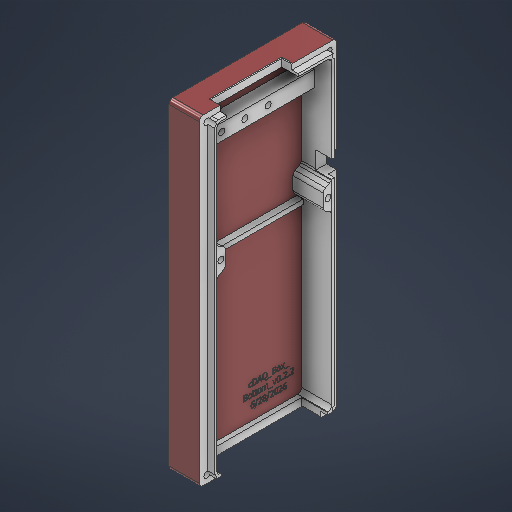
# Autodesk Inventor part: cDAQ_Box_Bottom_v0.2.3
Saved by Autodesk Inventor 2027 (Build 310192000, 192)
## iProperties
Created: 2026-05-08
Part Number: cDAQ_Box_Bottom_v0.2.3
Material: Generic
Document SubType Name: Modeling
Designer: giese
Density: 1 g/cm^3
Appearance: Default
Author: giese
Autodesk Inventor part; units mm, degrees
(part 1 of 2)
ref_plane "YZ Plane" through (0, 0, 0) normal (1, 0, 0) x (0, 1, 0)
ref_plane "XZ Plane" through (0, 0, 0) normal (0, 1, 0) x (-1, 0, 0)
ref_plane "XY Plane" through (0, 0, 0) normal (0, 0, 1) x (1, 0, 0)
sketch "Sketch1" plane through (0, 0, 0) normal (1, 0, 0) x (0, 1, 0)
  line L0 (37.5698, 60.7867) -> (-217.4462, 60.7867)
  line L1 (-217.4462, 60.7867) -> (-217.4462, -48.4333)
  line L2 (-217.4462, -48.4333) -> (37.5698, -48.4333)
  line L3 (37.5698, -48.4333) -> (37.5698, 60.7867)
  point P0 (0, 0)
  dimension "d0" = 109.22
  dimension "d1" = 255.016
  constraints: 8 end point, 2 parallel, 1 horizontal, 1 perpendicular
  measures "d0" distance of L2.end L0.start
  measures "d1" distance of L1.end L2.end
extrude "Extrusion1" add sketch "Sketch1" along normal blind 24.13
sketch "Sketch2" plane through (24.13, 0, 0) normal (1, 0, 0) x (0, 0, -1)
  line L0 (39.5433, 31.2198) -> (-51.8967, 31.2198)
  line L1 (-51.8967, 31.2198) -> (-51.8967, -211.0962)
  line L2 (-51.8967, -211.0962) -> (39.5433, -211.0962)
  line L3 (39.5433, -211.0962) -> (39.5433, 31.2198)
  line L4 (48.4333, 37.5698) -> (-60.7867, 37.5698) projected
  line L5 (-60.7867, 37.5698) -> (-60.7867, -217.4462) projected
  line L6 (-60.7867, -217.4462) -> (48.4333, -217.4462) projected
  line L7 (48.4333, -217.4462) -> (48.4333, 37.5698) projected
  point P0 (0, 0)
  dimension "d4" = 242.316
  dimension "d5" = 91.44
  dimension "d8" = 6.35
  dimension "d21" = 8.89
  dimension "d690" = 6.35
  dimension "d842" = 8.89
  constraints: 8 end point, 2 parallel, 1 horizontal, 1 perpendicular
  measures "d4" distance of L2.end L0.start
  measures "d5" distance of L0.start L0.end
  measures "d8" distance between parallel lines of L0 L4
  measures "d21" distance between parallel lines of L5 L1
  measures "d690" distance between parallel lines of L6 L2
  measures "d842" distance between parallel lines of L7 L3
extrude "Extrusion2" cut sketch "Sketch2" against normal blind 19.05 contours L3 L2 L1 L0
sketch "Sketch3" plane through (0, 0, 0) normal (-1, 0, 0) x (0, 0, 1)
  circle A0 centre (-2.8809, 9.6298) radius 2.4005
  circle A1 centre (15.6179, 9.6298) radius 2.4005
  circle A2 centre (34.1167, 9.6298) radius 2.4005
  line L0 (-48.4333, -217.4462) -> (-48.4333, 37.5698) projected
  line L1 (-48.4333, 37.5698) -> (60.7867, 37.5698) projected
  line L2 (60.7867, 37.5698) -> (60.7867, -217.4462) projected
  line L3 (51.8967, 31.2198) -> (-39.5433, 31.2198) projected
  point P0 (0, 0)
  point P1 (-0.896, -23.7433)
  point P2 (-45.1848, 27.0137)
  dimension "d9" = 18.4988
  dimension "d10" = 4.801
  dimension "d11" = 4.801
  dimension "d12" = 18.4988
  dimension "d13" = 36.9976
  dimension "d18" = 26.67
  dimension "d22" = 4.801
  dimension "d58" = 27.94
  constraints: 3 centre point
  measures "d9" distance of A0.centre A1.centre
  measures "d10" diameter of A1
  measures "d11" diameter of A2
  measures "d12" distance of A1.centre A2.centre
  measures "d13" distance of A0.centre A2.centre
  measures "d18" distance from line of L2 A2.centre
  measures "d22" diameter of A0
  measures "d58" distance from line of L1 A2.centre
extrude "Extrusion3" cut sketch "Sketch3" against normal blind 5.08
sketch "Sketch5" plane through (0, -217.4462, -48.4333) normal (0, 0, -1) x (-1, 0, 0)
  line L0 (-27.2034, 165.862) -> (-16.51, 165.862)
  line L1 (-16.51, 165.862) -> (-16.51, 178.562)
  line L2 (-16.51, 178.562) -> (-27.2034, 178.562)
  line L3 (-27.2034, 178.562) -> (-27.2034, 165.862)
  line L4 (0, 255.016) -> (-24.13, 255.016) projected
  line L5 (0, 0) -> (0, 255.016) projected
  line L6 (-24.13, 0) -> (-24.13, 255.016) projected
  line L7 (0, 0) -> (-24.13, 0) projected
  point P0 (0, 217.4462)
  point P1 (-21.8567, 178.562)
  point P2 (-21.8567, 165.862)
  dimension "d28" = 10.6934
  dimension "d30" = 12.7
  dimension "d31" = 16.51
  dimension "d215" = 3.0734
  dimension "d1133" = 165.862
  constraints: 8 end point, 2 midpoint, 2 parallel, 1 horizontal, 1 perpendicular
  measures "d28" distance between parallel lines of L1 L3
  measures "d30" distance of point (-21.857, 178.562) point (-21.857, 165.862)
  measures "d31" distance between parallel lines of L5 L1
  measures "d215" distance between parallel lines of L6 L3
  measures "d1133" distance between parallel lines of L7 L0
extrude "Extrusion4" cut sketch "Sketch5" against normal blind 24.13 contours L3 L2 L6 L0 | L6 L2 L1 L0
sketch "Sketch6" plane through (0, -217.4462, -48.4333) normal (0, -1, 0) x (1, 0, 0)
  line L0 (24.08, 55.136) -> (16.08, 55.136)
  line L1 (16.08, 45.136) -> (24.08, 45.136)
  line L2 (0, 109.22) -> (0, 0) projected
  line L3 (29.63, 53.1359) -> (29.63, 47.136)
  line L4 (24.08, 55.136) -> (29.63, 53.1359)
  line L5 (29.63, 47.136) -> (24.08, 45.136)
  line L6 (0, 0) -> (24.13, 0) projected
  line L7 (24.13, 100.33) -> (24.13, 8.89) projected
  line L8 (24.13, 41.9134) -> (24.13, 37.4697)
  line L9 (16.08, 55.136) -> (8.636, 55.136)
  line L10 (8.636, 55.136) -> (8.636, 45.136)
  line L11 (8.636, 45.136) -> (21.16, 45.136)
  point P0 (0, 48.4333)
  point P1 (20.08, 55.136)
  point P2 (20.08, 45.136)
  point P3 (16.08, 50.136)
  dimension "d39" = 6
  dimension "d48" = 55.136
  dimension "d221" = 0
  dimension "d223" = 2
  dimension "d224" = 2
  dimension "d225" = 5.5
  dimension "d227" = 5.55
  dimension "d672" = 8.636
  constraints: 18 end point, 2 horizontal, 2 midpoint, 2 parallel, 2 point on line, 1 perpendicular, 1 vertical
  measures "d39" distance of L3.start L3.end
  measures "d48" distance between parallel lines of L6 L0
  measures "d221" horizontal distance of L0.start L1.end
  measures "d223" vertical distance of L3.end L1.end
  measures "d224" vertical distance of L0.start L3.start
  measures "d225" distance between parallel lines of L3 L7
  measures "d227" distance from line of L1.end L3
  measures "d672" distance between parallel lines of L2 L10
extrude "Extrusion5" [suppressed]
sketch "Sketch7" plane through (0, 37.5698, 60.7867) normal (0, 1, 0) x (1, 0, 0)
  line L0 (31.0134, 73.66) -> (16.002, 73.66)
  line L1 (16.002, 73.66) -> (16.002, 16.51)
  line L2 (16.002, 16.51) -> (31.0134, 16.51)
  line L3 (31.0134, 16.51) -> (31.0134, 73.66)
  line L4 (0, 0) -> (24.13, 0) projected
  line L5 (0, 109.22) -> (0, 0) projected
  line L6 (24.13, 109.22) -> (24.13, 0) projected
  point P0 (0, 60.7867)
  point P1 (24.13, 73.66)
  point P2 (24.13, 16.51)
  dimension "d52" = 16.51
  dimension "d55" = 16.002
  dimension "d56" = 15.0114
  dimension "d57" = 6.8834
  dimension "d1702" = 57.15
  constraints: 8 end point, 2 parallel, 1 horizontal, 1 perpendicular
  measures "d52" distance between parallel lines of L4 L2
  measures "d55" distance between parallel lines of L5 L1
  measures "d56" distance between parallel lines of L3 L1
  measures "d57" distance between parallel lines of L6 L3
  measures "d1702" distance of L2.end L0.start
extrude "Extrusion6" cut sketch "Sketch7" against normal blind 7.62
fillet "Fillet1" radius 3.175 4 edges at (12.065, 37.5698, -48.4333) (12.065, 37.5698, 60.7867) (12.065, -217.4462, -48.4333) (12.065, -217.4462, 60.7867)
sketch "Sketch8" plane through (0, 0, 0) normal (-1, 0, 0) x (0, 0, 1)
  line L0 (13.7764, 5.9468) -> (17.4594, 5.9468)
  line L1 (13.7764, 13.3128) -> (17.4594, 13.3128)
  line L2 (13.7764, 5.9468) -> (11.65, 9.6298)
  line L3 (13.7764, 13.3128) -> (11.65, 9.6298)
  line L4 (17.4594, 5.9468) -> (19.5858, 9.6298)
  line L5 (17.4594, 13.3128) -> (19.5858, 9.6298)
  circle A0 centre (15.6179, 9.6298) radius 2.4005
  circle A1 centre (15.6179, 9.6298) radius 2.4005 projected
  line L6 (-1.0394, 13.3128) -> (1.0869, 9.6298)
  line L7 (-1.0394, 5.9468) -> (1.0869, 9.6298)
  line L8 (-4.7224, 13.3128) -> (-1.0394, 13.3128)
  line L9 (-4.7224, 5.9468) -> (-1.0394, 5.9468)
  circle A2 centre (-2.8809, 9.6298) radius 2.4005
  line L10 (-4.7224, 13.3128) -> (-6.8488, 9.6298)
  line L11 (-4.7224, 5.9468) -> (-6.8488, 9.6298)
  circle A3 centre (-2.8809, 9.6298) radius 2.4005
  circle A4 centre (-2.8809, 9.6298) radius 2.4005 projected
  line L12 (35.9582, 13.3128) -> (38.0846, 9.6298)
  line L13 (35.9582, 5.9468) -> (38.0846, 9.6298)
  line L14 (32.2752, 13.3128) -> (35.9582, 13.3128)
  line L15 (32.2752, 5.9468) -> (35.9582, 5.9468)
  circle A5 centre (34.1167, 9.6298) radius 2.4005
  line L16 (32.2752, 13.3128) -> (30.1488, 9.6298)
  line L17 (32.2752, 5.9468) -> (30.1488, 9.6298)
  circle A6 centre (34.1167, 9.6298) radius 2.4005
  circle A7 centre (34.1167, 9.6298) radius 2.4005 projected
  point P0 (15.6179, 5.9468)
  point P1 (-2.8809, 5.9468)
  point P2 (34.1167, 5.9468)
  point P3 (1.0869, 9.6298)
  dimension "d1514" = 120
  dimension "d1515" = 120
  dimension "d1516" = 120
  dimension "d1517" = 120
  dimension "d1518" = 3.683
  dimension "d1519" = 3.683
  dimension "d1520" = 3.683
  dimension "d1521" = 3.683
  dimension "d1522" = 0
  dimension "d1523" = 3.683
  dimension "d1524" = 0
  dimension "d1525" = 3.683
  dimension "d1526" = 1.8415
  dimension "d1527" = 7.366
  dimension "d1528" = 7.9358
  dimension "d1529" = 0
  dimension "d1530" = 0
  dimension "d1531" = 7.9358
  dimension "d1532" = 0
  dimension "d1710" = 120
  dimension "d1711" = 120
  dimension "d1712" = 120
  dimension "d1713" = 120
  dimension "d1714" = 3.683
  dimension "d1715" = 3.683
  dimension "d1716" = 3.683
  dimension "d1717" = 3.683
  dimension "d1718" = 0
  dimension "d1719" = 3.683
  dimension "d1720" = 0
  dimension "d1721" = 3.683
  dimension "d1722" = 1.8415
  dimension "d1723" = 7.366
  dimension "d1724" = 7.9358
  dimension "d1725" = 0
  dimension "d1726" = 0
  dimension "d1727" = 7.9358
  dimension "d1728" = 0
  dimension "d1729" = 0
  dimension "d1730" = 0
  dimension "d1731" = 120
  dimension "d1732" = 120
  dimension "d1733" = 120
  dimension "d1734" = 120
  dimension "d1735" = 3.683
  dimension "d1736" = 3.683
  dimension "d1737" = 3.683
  dimension "d1738" = 3.683
  dimension "d1739" = 0
  dimension "d1740" = 3.683
  dimension "d1741" = 0
  dimension "d1742" = 3.683
  dimension "d1743" = 1.8415
  dimension "d1744" = 7.366
  dimension "d1745" = 7.9358
  dimension "d1746" = 0
  dimension "d1747" = 0
  dimension "d1748" = 7.9358
  dimension "d1749" = 0
  dimension "d1750" = 0
  dimension "d1751" = 0
  constraints: 36 end point, 6 horizontal, 5 centre point, 3 midpoint
  measures "d1514" angle of L0 L2
  measures "d1515" angle of L1 L3
  measures "d1516" angle of L4 L0
  measures "d1517" angle of L5 L1
  measures "d1518" distance of L0.start L4.start
  measures "d1519" distance of L1.start L5.start
  measures "d1520" vertical distance of L4.start L4.end
  measures "d1521" vertical distance of L3.end L1.start
  measures "d1522" vertical distance of A0.centre L3.end
  measures "d1523" vertical distance of L2.end L0.start
  measures "d1524" vertical distance of A0.centre L2.end
  measures "d1525" vertical distance of L5.end L5.start
  measures "d1526" horizontal distance of A0.centre L5.start
  measures "d1527" distance of L4.start L5.start
  measures "d1528" distance of L3.end L5.end
  measures "d1529" distance of A1.centre A0.centre
  measures "d1530" distance of A1.centre A0.centre
  measures "d1531" distance of L4.end L2.end
  measures "d1532" distance of L3.end L2.end
  measures "d1710" angle of L9 L11
  measures "d1711" angle of L8 L10
  measures "d1712" angle of L7 L9
  measures "d1713" angle of L6 L8
  measures "d1714" distance of L9.start L9.end
  measures "d1715" distance of L10.start L6.start
  measures "d1716" vertical distance of L9.end L7.end
  measures "d1717" vertical distance of L10.end L10.start
  measures "d1718" vertical distance of A2.centre L10.end
  measures "d1719" vertical distance of L11.end L9.start
  measures "d1720" vertical distance of A2.centre L11.end
  measures "d1721" vertical distance of L6.end L6.start
  measures "d1722" horizontal distance of A2.centre L6.start
  measures "d1723" distance of L9.end L6.start
  measures "d1724" distance of L10.end L6.end
  measures "d1725" distance of A3.centre A2.centre
  measures "d1726" distance of A3.centre A2.centre
  measures "d1727" distance of L7.end L11.end
  measures "d1728" distance of L10.end L11.end
  measures "d1729" distance of A4.centre A2.centre
  measures "d1730" distance of A4.centre A3.centre
  measures "d1731" angle of L15 L17
  measures "d1732" angle of L14 L16
  measures "d1733" angle of L13 L15
  measures "d1734" angle of L12 L14
  measures "d1735" distance of L17.start L13.start
  measures "d1736" distance of L16.start L12.start
  measures "d1737" vertical distance of L13.start L13.end
  measures "d1738" vertical distance of L16.end L16.start
  measures "d1739" vertical distance of A5.centre L16.end
  measures "d1740" vertical distance of L17.end L17.start
  measures "d1741" vertical distance of A5.centre L17.end
  measures "d1742" vertical distance of L12.end L12.start
  measures "d1743" horizontal distance of A5.centre L12.start
  measures "d1744" distance of L13.start L12.start
  measures "d1745" distance of L16.end L12.end
  measures "d1746" distance of A6.centre A5.centre
  measures "d1747" distance of A6.centre A5.centre
  measures "d1748" distance of L13.end L17.end
  measures "d1749" distance of L16.end L17.end
  measures "d1750" distance of A7.centre A5.centre
  measures "d1751" distance of A7.centre A5.centre
extrude "Extrusion7" cut sketch "Sketch8" against normal blind 5
sketch "Sketch9" plane through (5.08, 0, 0) normal (1, 0, 0) x (0, 0, -1)
  arc A0 (22.2689, -180.8044) -> (16.8127, -180.8044) centre (19.5408, -178.3302) ccw
  line L0 (45.2583, 37.5698) -> (12.8733, 37.5698) projected
  line L1 (39.5433, 31.2198) -> (39.5433, -38.8842) projected
  arc A1 (17.6358, -185.9502) -> (21.4458, -185.9502) centre (19.5408, -185.9502) ccw
  line L2 (21.4458, -185.9502) -> (21.4458, -182.9374)
  line L3 (17.6358, -185.9502) -> (17.6358, -182.9374)
  arc A2 (22.2689, -180.8044) -> (21.4458, -182.9374) centre (24.6208, -182.9374) ccw
  arc A3 (17.6358, -182.9374) -> (16.8127, -180.8044) centre (14.4608, -182.9374) ccw
  arc A4 (-28.5311, -180.8044) -> (-33.9873, -180.8045) centre (-31.2592, -178.3302) ccw
  arc A5 (-33.1642, -185.9366) -> (-29.3542, -185.9502) centre (-31.2592, -185.9502) ccw
  line L4 (-29.3542, -185.9502) -> (-29.3542, -182.9374)
  line L5 (-33.1642, -185.9366) -> (-33.1642, -182.9374)
  arc A6 (-28.5311, -180.8044) -> (-29.3542, -182.9374) centre (-26.1792, -182.9374) ccw
  arc A7 (-33.1642, -182.9374) -> (-33.9873, -180.8045) centre (-36.3392, -182.9374) ccw
  line L6 (-44.2767, 37.5698) -> (-57.6117, 37.5698) projected
  line L7 (-51.8967, -211.0962) -> (-51.8967, 31.2198) projected
  point P0 (0, 0)
  point P1 (39.5433, -211.0962)
  point P2 (21.4458, -181.4823)
  point P3 (17.6358, -181.4823)
  point P4 (-29.3542, -181.4823)
  point P5 (-33.1642, -181.4823)
  point P6 (-51.8967, 31.2198)
  point P7 (-49.3567, -207.2862)
  dimension "d112" = 215.9
  dimension "d114" = 7.366
  dimension "d116" = 3.81
  dimension "d117" = 223.52
  dimension "d118" = 3.175
  dimension "d119" = 7.366
  dimension "d120" = 3.81
  dimension "d121" = 3.175
  dimension "d122" = 215.9
  dimension "d123" = 223.52
  dimension "d125" = 0
  dimension "d128" = 50.8
  dimension "d129" = 20.0025
  dimension "d130" = 0
  constraints: 20 point on circle, 8 centre point, 8 end point, 8 tangent, 4 point on line, 2 equal radius, 2 parallel, 2 vertical, 1 other
  measures "d112" distance from line of L0 A0.centre
  measures "d114" diameter of A0
  measures "d116" diameter of A1
  measures "d117" distance from line of L0 A1.centre
  measures "d118" radius of A2
  measures "d119" diameter of A4
  measures "d120" diameter of A5
  measures "d121" radius of A6
  measures "d122" distance from line of A4.centre L6
  measures "d123" distance from line of L6 A5.centre
  measures "d125" horizontal distance of A5.centre A4.centre
  measures "d128" distance of A5.centre A1.centre
  measures "d129" distance from line of L1 A0.centre
  measures "d130" horizontal distance of A0.centre A1.centre
extrude "Extrusion8" [suppressed]
sketch "Sketch10" plane through (24.13, 0, 0) normal (1, 0, 0) x (0, 0, -1)
  line L0 (-51.8967, 31.2198) -> (39.5433, 31.2198) projected
  line L1 (-51.8967, 31.2198) -> (39.5433, 31.2198)
  line L2 (42.0833, 33.2264) -> (-46.8167, 33.2264)
  line L3 (-46.8167, 33.2264) -> (-53.9033, 33.2264)
  line L4 (-53.9033, 33.2264) -> (-53.9033, -213.1028)
  line L5 (-53.9033, -213.1028) -> (41.5499, -213.1028)
  line L6 (41.5499, -213.1028) -> (41.5499, 33.2264)
  line L7 (41.5499, 33.2264) -> (41.9392, 33.2264)
  line L8 (39.5433, 31.2198) -> (39.5433, -38.8842) projected
  line L9 (-51.8967, -211.0962) -> (-51.8967, 31.2198) projected
  line L10 (39.5433, -211.0962) -> (-51.8967, -211.0962) projected
  line L11 (45.2583, 37.5698) -> (12.8733, 37.5698) projected
  line L12 (39.5433, 31.2198) -> (39.5433, -211.0962)
  line L13 (39.5433, -211.0962) -> (-51.8967, -211.0962)
  line L14 (-57.6117, -217.4462) -> (45.2583, -217.4462) projected
  line L15 (-51.8967, -211.0962) -> (-51.8967, 31.2198)
  line L16 (-51.8967, 31.2198) -> (39.5433, 31.2198)
  line L17 (-51.8967, 31.2198) -> (39.5433, 31.2198)
  line L18 (39.5433, 31.2198) -> (39.5433, -211.0962)
  line L19 (39.5433, -211.0962) -> (-51.8967, -211.0962)
  line L20 (-51.8967, -211.0962) -> (-51.8967, 31.2198)
  point P0 (41.5499, 33.2264)
  point P1 (-49.3567, -207.2862)
  point P2 (39.5433, -38.8842)
  dimension "d202" = 2.0066
  dimension "d203" = 2.0066
  dimension "d204" = 2.0066
  dimension "d205" = 2.0066
  dimension "d208" = 4.3434
  constraints: 30 end point, 6 perpendicular, 3 collinear, 3 point on line, 2 horizontal, 2 parallel, 2 other
  measures "d202" distance between parallel lines of L0 L2
  measures "d203" distance between parallel lines of L6 L8
  measures "d205" distance between parallel lines of L5 L10
  measures "d208" distance between parallel lines of L11 L2
extrude "Extrusion9" add sketch "Sketch10" along normal blind 5
fillet "Fillet2" radius 3.175 7 edges at (17.105, 31.2198, -39.5433) (17.105, 31.2198, 51.8967) (17.105, -211.0962, 51.8967) (17.105, -211.0962, -39.5433) (26.63, 33.2264, 53.9033) (26.63, -213.1028, -41.5499) (26.63, -213.1028, 53.9033)
sketch "Sketch13" plane through (29.13, 0, 0) normal (1, 0, 0) x (0, 0, -1)
  arc A0 (44.0833, 30.0448) -> (40.9083, 33.2198) centre (40.9083, 30.0448) ccw projected
  arc A1 (-45.6417, 33.2198) -> (-48.8167, 30.0448) centre (-45.6417, 30.0448) ccw projected
  arc A2 (40.9083, -212.0802) -> (44.0833, -208.9052) centre (40.9083, -208.9052) ccw projected
  arc A3 (-48.8167, -208.9052) -> (-45.6417, -212.0802) centre (-45.6417, -208.9052) ccw projected
  line L0 (-44.2767, 37.5698) -> (-57.6117, 37.5698) projected
  line L1 (-60.7867, 34.3948) -> (-60.7867, -214.2712) projected
  line L2 (-57.6117, -217.4462) -> (45.2583, -217.4462) projected
  arc A4 (-48.8167, -208.9052) -> (-45.6417, -212.0802) centre (-45.6417, -208.9052) ccw projected
  circle A5 centre (-54.6907, -211.3502) radius 2.4005
  circle A6 centre (42.3373, -211.3502) radius 2.4005
  line L3 (48.4333, -214.2712) -> (48.4333, 34.3948) projected
  circle A7 centre (42.3373, 31.4738) radius 2.4005
  line L4 (45.2583, 37.5698) -> (12.8733, 37.5698) projected
  circle A8 centre (-54.6907, 31.4738) radius 2.4005
  arc A9 (41.4904, -28.6131) -> (38.3154, -25.4381) centre (38.3154, -28.6131) ccw
  circle A10 centre (36.3683, -64.0302) radius 2.4005
  circle A11 centre (-48.7217, -64.0302) radius 2.4005
  point P0 (0, 0)
  point P1 (-47.8868, 32.2898)
  point P2 (-47.8868, -211.1503)
  point P3 (-47.8868, -211.1503)
  point P4 (45.8404, -24.2631)
  point P5 (42.6654, -21.0881)
  dimension "d178" = 6.096
  dimension "d179" = 6.096
  dimension "d180" = 4.801
  dimension "d181" = 6.096
  dimension "d182" = 6.096
  dimension "d183" = 4.801
  dimension "d184" = 4.801
  dimension "d185" = 6.096
  dimension "d186" = 6.096
  dimension "d187" = 4.801
  dimension "d188" = 6.096
  dimension "d189" = 6.096
  dimension "d326" = 4.801
  dimension "d327" = 12.065
  dimension "d328" = 101.6
  dimension "d329" = 4.801
  dimension "d330" = 12.065
  dimension "d331" = 101.6
  constraints: 7 centre point, 5 point on circle
  measures "d178" distance from line of L1 A5.centre
  measures "d179" distance from line of L2 A5.centre
  measures "d180" diameter of A5
  measures "d181" distance from line of L2 A6.centre
  measures "d182" distance from line of L3 A6.centre
  measures "d183" diameter of A6
  measures "d184" diameter of A7
  measures "d185" distance from line of L3 A7.centre
  measures "d186" distance from line of L4 A7.centre
  measures "d187" diameter of A8
  measures "d188" distance from line of L0 A8.centre
  measures "d189" distance from line of L1 A8.centre
  measures "d326" diameter of A10
  measures "d327" distance from line of L3 A10.centre
  measures "d328" distance from line of A10.centre L4
  measures "d329" diameter of A11
  measures "d330" distance from line of L1 A11.centre
  measures "d331" distance from line of L0 A11.centre
extrude "Extrusion11" cut sketch "Sketch13" against normal blind 25.4
sketch "Sketch14" plane through (5.08, 0, 0) normal (1, 0, 0) x (0, 0, -1)
  line L0 (3.8756, -183.0595) -> (23.0923, -183.0595) construction
  line L1 (23.0923, -183.0595) -> (23.0923, -181.11) construction
  line L2 (23.0923, -181.11) -> (3.8756, -181.11) construction
  line L3 (3.8756, -181.11) -> (3.8756, -183.0595) construction
  spline S0 degree 2 poles (-1.0212, -187.8056) (-1.3769, -187.8056) (-1.966, -187.587) (-2.1772, -187.3647) knots 0 0 0 1 2 2 2
  spline S1 degree 2 poles (-2.1772, -187.3647) (-2.3884, -187.1461) (-2.6218, -186.4718) (-2.6218, -186.0198) knots 0 0 0 1 2 2 2
  spline S2 degree 2 poles (-2.6218, -186.0198) (-2.6218, -185.5678) (-2.381, -184.9083) (-2.1772, -184.686) knots 0 0 0 1 2 2 2
  spline S3 degree 2 poles (-2.1772, -184.686) (-1.9734, -184.46) (-1.3695, -184.2192) (-1.0212, -184.2192) knots 0 0 0 1 2 2 2
  spline S4 degree 2 poles (-1.0212, -184.2192) (-0.7396, -184.2192) (-0.2135, -184.3785) (-0.0097, -184.4822) knots 0 0 0 1 2 2 2
  line L4 (-0.0097, -184.4822) -> (-0.0097, -185.1306)
  line L5 (-0.0097, -185.1306) -> (-0.0431, -185.1306)
  spline S5 degree 2 poles (-0.0431, -185.1306) (-0.1061, -185.0787) (-0.2987, -184.9453) (-0.4358, -184.875) knots 0 0 0 1 2 2 2
  spline S6 degree 2 poles (-0.4358, -184.875) (-0.5581, -184.8157) (-0.8841, -184.723) (-1.0323, -184.723) knots 0 0 0 1 2 2 2
  spline S7 degree 2 poles (-1.0323, -184.723) (-1.4806, -184.723) (-2.0253, -185.4011) (-2.0253, -186.0198) knots 0 0 0 1 2 2 2
  spline S8 degree 2 poles (-2.0253, -186.0198) (-2.0253, -186.6237) (-1.4992, -187.3017) (-1.0323, -187.3017) knots 0 0 0 1 2 2 2
  spline S9 degree 2 poles (-1.0323, -187.3017) (-0.7507, -187.3017) (-0.2395, -187.0683) (-0.0431, -186.8868) knots 0 0 0 1 2 2 2
  line L6 (-0.0431, -186.8868) -> (-0.0097, -186.8868)
  line L7 (-0.0097, -186.8868) -> (-0.0097, -187.5352)
  spline S10 degree 2 poles (-0.0097, -187.5352) (-0.095, -187.5759) (-0.3543, -187.6908) (-0.4581, -187.7167) knots 0 0 0 1 2 2 2
  spline S11 degree 2 poles (-0.4581, -187.7167) (-0.6063, -187.7612) (-0.8397, -187.8056) (-1.0212, -187.8056) knots 0 0 0 1 2 2 2
  spline S12 degree 2 poles (4.1658, -185.4455) (4.1658, -186.0717) (3.6582, -187.0794) (3.2322, -187.361) knots 0 0 0 1 2 2 2
  spline S13 degree 2 poles (3.2322, -187.361) (2.8839, -187.5796) (2.1688, -187.7278) (1.6131, -187.7278) knots 0 0 0 1 2 2 2
  line L8 (1.6131, -187.7278) -> (0.5608, -187.7278)
  line L9 (0.5608, -187.7278) -> (0.5608, -183.1558)
  line L10 (0.5608, -183.1558) -> (1.6019, -183.1558)
  spline S14 degree 2 poles (1.6019, -183.1558) (2.2466, -183.1558) (2.9802, -183.3485) (3.2396, -183.5189) knots 0 0 0 1 2 2 2
  spline S15 degree 2 poles (3.2396, -183.5189) (3.6805, -183.8116) (4.1658, -184.7786) (4.1658, -185.4455) knots 0 0 0 1 2 2 2
  spline S16 degree 2 poles (3.5323, -185.4381) (3.5323, -184.912) (3.184, -184.1673) (2.8394, -183.9561) knots 0 0 0 1 2 2 2
  spline S17 degree 2 poles (2.8394, -183.9561) (2.5949, -183.8116) (2.0428, -183.6819) (1.6316, -183.6819) knots 0 0 0 1 2 2 2
  line L11 (1.6316, -183.6819) -> (1.1685, -183.6819)
  line L12 (1.1685, -183.6819) -> (1.1685, -187.2017)
  line L13 (1.1685, -187.2017) -> (1.6316, -187.2017)
  spline S18 degree 2 poles (1.6316, -187.2017) (2.0354, -187.2017) (2.6468, -187.072) (2.895, -186.8979) knots 0 0 0 1 2 2 2
  spline S19 degree 2 poles (2.895, -186.8979) (3.2136, -186.683) (3.5323, -185.9716) (3.5323, -185.4381) knots 0 0 0 1 2 2 2
  line L14 (4.3325, -187.7278) -> (5.8738, -183.1558)
  line L15 (5.8738, -183.1558) -> (6.6222, -183.1558)
  line L16 (6.6222, -183.1558) -> (8.1635, -187.7278)
  line L17 (8.1635, -187.7278) -> (7.5226, -187.7278)
  line L18 (7.5226, -187.7278) -> (7.1076, -186.4496)
  line L19 (7.1076, -186.4496) -> (5.3625, -186.4496)
  line L20 (5.3625, -186.4496) -> (4.9476, -187.7278)
  line L21 (4.9476, -187.7278) -> (4.3325, -187.7278)
  line L22 (6.9409, -185.9309) -> (6.2332, -183.7783)
  line L23 (6.2332, -183.7783) -> (5.5293, -185.9309)
  line L24 (5.5293, -185.9309) -> (6.9409, -185.9309)
  spline S20 degree 2 poles (12.3947, -188.8467) (12.228, -188.8875) (11.8649, -188.932) (11.6833, -188.932) knots 0 0 0 1 2 2 2
  spline S21 degree 2 poles (11.6833, -188.932) (11.1683, -188.932) (10.5273, -188.3577) (10.4977, -187.8242) knots 0 0 0 1 2 2 2
  spline S22 degree 2 poles (10.4977, -187.8242) (10.4569, -187.8242) (10.3866, -187.8242) (10.3569, -187.8242) knots 0 0 0 1 2 2 2
  spline S23 degree 2 poles (10.3569, -187.8242) (9.8938, -187.8242) (9.1491, -187.5092) (8.8823, -187.2017) knots 0 0 0 1 2 2 2
  spline S24 degree 2 poles (8.8823, -187.2017) (8.6193, -186.8979) (8.3377, -186.0087) (8.3377, -185.4455) knots 0 0 0 1 2 2 2
  spline S25 degree 2 poles (8.3377, -185.4455) (8.3377, -184.8675) (8.623, -183.9932) (8.886, -183.6819) knots 0 0 0 1 2 2 2
  spline S26 degree 2 poles (8.886, -183.6819) (9.1528, -183.3744) (9.8975, -183.0595) (10.3569, -183.0595) knots 0 0 0 1 2 2 2
  spline S27 degree 2 poles (10.3569, -183.0595) (10.8237, -183.0595) (11.5722, -183.3855) (11.8315, -183.6819) knots 0 0 0 1 2 2 2
  spline S28 degree 2 poles (11.8315, -183.6819) (12.0909, -183.982) (12.3799, -184.875) (12.3799, -185.4455) knots 0 0 0 1 2 2 2
  spline S29 degree 2 poles (12.3799, -185.4455) (12.3799, -186.3347) (11.687, -187.4907) (11.0831, -187.6945) knots 0 0 0 1 2 2 2
  spline S30 degree 2 poles (11.0831, -187.6945) (11.0979, -187.8649) (11.1868, -188.1391) (11.2572, -188.2169) knots 0 0 0 1 2 2 2
  spline S31 degree 2 poles (11.2572, -188.2169) (11.3424, -188.3132) (11.5759, -188.4021) (11.7833, -188.4021) knots 0 0 0 1 2 2 2
  spline S32 degree 2 poles (11.7833, -188.4021) (11.9056, -188.4021) (12.2391, -188.3243) (12.3132, -188.2947) knots 0 0 0 1 2 2 2
  line L25 (12.3132, -188.2947) -> (12.3947, -188.2947)
  line L26 (12.3947, -188.2947) -> (12.3947, -188.8467)
  spline S33 degree 2 poles (11.7463, -185.4455) (11.7463, -184.9898) (11.5499, -184.2896) (11.3721, -184.0598) knots 0 0 0 1 2 2 2
  spline S34 degree 2 poles (11.3721, -184.0598) (11.1905, -183.8227) (10.6793, -183.5856) (10.3606, -183.5856) knots 0 0 0 1 2 2 2
  spline S35 degree 2 poles (10.3606, -183.5856) (10.0309, -183.5856) (9.5344, -183.8153) (9.3454, -184.0598) knots 0 0 0 1 2 2 2
  spline S36 degree 2 poles (9.3454, -184.0598) (9.1639, -184.2933) (8.9712, -185.0009) (8.9712, -185.4455) knots 0 0 0 1 2 2 2
  spline S37 degree 2 poles (8.9712, -185.4455) (8.9712, -186.3458) (9.7271, -187.3054) (10.3606, -187.3054) knots 0 0 0 1 2 2 2
  spline S38 degree 2 poles (10.3606, -187.3054) (10.9942, -187.3054) (11.7463, -186.3458) (11.7463, -185.4455) knots 0 0 0 1 2 2 2
  line L27 (16.0627, -188.6467) -> (12.5355, -188.6467)
  line L28 (12.5355, -188.6467) -> (12.5355, -188.2502)
  line L29 (12.5355, -188.2502) -> (16.0627, -188.2502)
  line L30 (16.0627, -188.2502) -> (16.0627, -188.6467)
  spline S39 degree 2 poles (19.5787, -186.3236) (19.5787, -186.6645) (19.3194, -187.1869) (19.1045, -187.3573) knots 0 0 0 1 2 2 2
  spline S40 degree 2 poles (19.1045, -187.3573) (18.8451, -187.5574) (18.256, -187.7278) (17.7892, -187.7278) knots 0 0 0 1 2 2 2
  line L31 (17.7892, -187.7278) -> (16.4776, -187.7278)
  line L32 (16.4776, -187.7278) -> (16.4776, -183.1558)
  line L33 (16.4776, -183.1558) -> (17.6892, -183.1558)
  spline S41 degree 2 poles (17.6892, -183.1558) (18.1782, -183.1558) (18.6673, -183.2188) (18.8896, -183.3411) knots 0 0 0 1 2 2 2
  spline S42 degree 2 poles (18.8896, -183.3411) (19.1378, -183.4707) (19.3638, -183.8968) (19.3638, -184.1858) knots 0 0 0 1 2 2 2
  spline S43 degree 2 poles (19.3638, -184.1858) (19.3638, -184.5082) (19.023, -185.0194) (18.7229, -185.1639) knots 0 0 0 1 2 2 2
  line L34 (18.7229, -185.1639) -> (18.7229, -185.1862)
  spline S44 degree 2 poles (18.7229, -185.1862) (19.1304, -185.2973) (19.5787, -185.8864) (19.5787, -186.3236) knots 0 0 0 1 2 2 2
  spline S45 degree 2 poles (18.9452, -186.3496) (18.9452, -186.0902) (18.797, -185.7567) (18.5747, -185.6382) knots 0 0 0 1 2 2 2
  spline S46 degree 2 poles (18.5747, -185.6382) (18.4302, -185.5641) (18.0893, -185.5196) (17.7744, -185.5196) knots 0 0 0 1 2 2 2
  line L35 (17.7744, -185.5196) -> (17.0852, -185.5196)
  line L36 (17.0852, -185.5196) -> (17.0852, -187.2091)
  line L37 (17.0852, -187.2091) -> (17.578, -187.2091)
  spline S47 degree 2 poles (17.578, -187.2091) (17.9781, -187.2091) (18.4376, -187.135) (18.6154, -187.0165) knots 0 0 0 1 2 2 2
  spline S48 degree 2 poles (18.6154, -187.0165) (18.7858, -186.8942) (18.9452, -186.5904) (18.9452, -186.3496) knots 0 0 0 1 2 2 2
  spline S49 degree 2 poles (18.7303, -184.271) (18.7303, -184.108) (18.6191, -183.8635) (18.4969, -183.7931) knots 0 0 0 1 2 2 2
  spline S50 degree 2 poles (18.4969, -183.7931) (18.3487, -183.7116) (17.9893, -183.6745) (17.6669, -183.6745) knots 0 0 0 1 2 2 2
  line L38 (17.6669, -183.6745) -> (17.0852, -183.6745)
  line L39 (17.0852, -183.6745) -> (17.0852, -185.012)
  line L40 (17.0852, -185.012) -> (17.7744, -185.012)
  spline S51 degree 2 poles (17.7744, -185.012) (18.0597, -185.012) (18.3301, -184.9528) (18.4746, -184.8601) knots 0 0 0 1 2 2 2
  spline S52 degree 2 poles (18.4746, -184.8601) (18.6154, -184.7712) (18.7303, -184.4859) (18.7303, -184.271) knots 0 0 0 1 2 2 2
  spline S53 degree 2 poles (22.9577, -186.0124) (22.9577, -186.8794) (22.1241, -187.8242) (21.4275, -187.8242) knots 0 0 0 1 2 2 2
  spline S54 degree 2 poles (21.4275, -187.8242) (20.7125, -187.8242) (19.8936, -186.8497) (19.8936, -186.0124) knots 0 0 0 1 2 2 2
  spline S55 degree 2 poles (19.8936, -186.0124) (19.8936, -185.1528) (20.7384, -184.2006) (21.4275, -184.2006) knots 0 0 0 1 2 2 2
  spline S56 degree 2 poles (21.4275, -184.2006) (22.1241, -184.2006) (22.9577, -185.1491) (22.9577, -186.0124) knots 0 0 0 1 2 2 2
  spline S57 degree 2 poles (22.3612, -186.0124) (22.3612, -185.3455) (21.8758, -184.6971) (21.4275, -184.6971) knots 0 0 0 1 2 2 2
  spline S58 degree 2 poles (21.4275, -184.6971) (20.9792, -184.6971) (20.4902, -185.3455) (20.4902, -186.0124) knots 0 0 0 1 2 2 2
  spline S59 degree 2 poles (20.4902, -186.0124) (20.4902, -186.6608) (20.9792, -187.3277) (21.4275, -187.3277) knots 0 0 0 1 2 2 2
  spline S60 degree 2 poles (21.4275, -187.3277) (21.8721, -187.3277) (22.3612, -186.6719) (22.3612, -186.0124) knots 0 0 0 1 2 2 2
  line L41 (26.2144, -187.7278) -> (25.5068, -187.7278)
  line L42 (25.5068, -187.7278) -> (24.6731, -186.4385)
  line L43 (24.6731, -186.4385) -> (23.8173, -187.7278)
  line L44 (23.8173, -187.7278) -> (23.1615, -187.7278)
  line L45 (23.1615, -187.7278) -> (24.3508, -186.0272)
  line L46 (24.3508, -186.0272) -> (23.1726, -184.297)
  line L47 (23.1726, -184.297) -> (23.8803, -184.297)
  line L48 (23.8803, -184.297) -> (24.7102, -185.5752)
  line L49 (24.7102, -185.5752) -> (25.5586, -184.297)
  line L50 (25.5586, -184.297) -> (26.2144, -184.297)
  line L51 (26.2144, -184.297) -> (25.0325, -185.9902)
  line L52 (25.0325, -185.9902) -> (26.2144, -187.7278)
  line L53 (29.7231, -188.6467) -> (26.1959, -188.6467)
  line L54 (26.1959, -188.6467) -> (26.1959, -188.2502)
  line L55 (26.1959, -188.2502) -> (29.7231, -188.2502)
  line L56 (29.7231, -188.2502) -> (29.7231, -188.6467)
  spline S61 degree 2 poles (-3.2924, -193.8513) (-3.2924, -194.1922) (-3.5517, -194.7146) (-3.7666, -194.885) knots 0 0 0 1 2 2 2
  spline S62 degree 2 poles (-3.7666, -194.885) (-4.026, -195.0851) (-4.6151, -195.2555) (-5.0819, -195.2555) knots 0 0 0 1 2 2 2
  line L57 (-5.0819, -195.2555) -> (-6.3935, -195.2555)
  line L58 (-6.3935, -195.2555) -> (-6.3935, -190.6835)
  line L59 (-6.3935, -190.6835) -> (-5.182, -190.6835)
  spline S63 degree 2 poles (-5.182, -190.6835) (-4.6929, -190.6835) (-4.2038, -190.7465) (-3.9815, -190.8687) knots 0 0 0 1 2 2 2
  spline S64 degree 2 poles (-3.9815, -190.8687) (-3.7333, -190.9984) (-3.5073, -191.4245) (-3.5073, -191.7135) knots 0 0 0 1 2 2 2
  spline S65 degree 2 poles (-3.5073, -191.7135) (-3.5073, -192.0358) (-3.8482, -192.5471) (-4.1483, -192.6916) knots 0 0 0 1 2 2 2
  line L60 (-4.1483, -192.6916) -> (-4.1483, -192.7139)
  spline S66 degree 2 poles (-4.1483, -192.7139) (-3.7407, -192.825) (-3.2924, -193.4141) (-3.2924, -193.8513) knots 0 0 0 1 2 2 2
  spline S67 degree 2 poles (-3.926, -193.8772) (-3.926, -193.6179) (-4.0742, -193.2844) (-4.2965, -193.1659) knots 0 0 0 1 2 2 2
  spline S68 degree 2 poles (-4.2965, -193.1659) (-4.441, -193.0918) (-4.7818, -193.0473) (-5.0967, -193.0473) knots 0 0 0 1 2 2 2
  line L61 (-5.0967, -193.0473) -> (-5.7859, -193.0473)
  line L62 (-5.7859, -193.0473) -> (-5.7859, -194.7368)
  line L63 (-5.7859, -194.7368) -> (-5.2931, -194.7368)
  spline S69 degree 2 poles (-5.2931, -194.7368) (-4.893, -194.7368) (-4.4335, -194.6627) (-4.2557, -194.5441) knots 0 0 0 1 2 2 2
  spline S70 degree 2 poles (-4.2557, -194.5441) (-4.0853, -194.4219) (-3.926, -194.1181) (-3.926, -193.8772) knots 0 0 0 1 2 2 2
  spline S71 degree 2 poles (-4.1408, -191.7987) (-4.1408, -191.6357) (-4.252, -191.3912) (-4.3743, -191.3208) knots 0 0 0 1 2 2 2
  spline S72 degree 2 poles (-4.3743, -191.3208) (-4.5225, -191.2393) (-4.8819, -191.2022) (-5.2042, -191.2022) knots 0 0 0 1 2 2 2
  line L64 (-5.2042, -191.2022) -> (-5.7859, -191.2022)
  line L65 (-5.7859, -191.2022) -> (-5.7859, -192.5397)
  line L66 (-5.7859, -192.5397) -> (-5.0967, -192.5397)
  spline S73 degree 2 poles (-5.0967, -192.5397) (-4.8115, -192.5397) (-4.541, -192.4804) (-4.3965, -192.3878) knots 0 0 0 1 2 2 2
  spline S74 degree 2 poles (-4.3965, -192.3878) (-4.2557, -192.2989) (-4.1408, -192.0136) (-4.1408, -191.7987) knots 0 0 0 1 2 2 2
  spline S75 degree 2 poles (0.0866, -193.5401) (0.0866, -194.407) (-0.747, -195.3518) (-1.4436, -195.3518) knots 0 0 0 1 2 2 2
  spline S76 degree 2 poles (-1.4436, -195.3518) (-2.1587, -195.3518) (-2.9775, -194.3774) (-2.9775, -193.5401) knots 0 0 0 1 2 2 2
  spline S77 degree 2 poles (-2.9775, -193.5401) (-2.9775, -192.6805) (-2.1327, -191.7283) (-1.4436, -191.7283) knots 0 0 0 1 2 2 2
  spline S78 degree 2 poles (-1.4436, -191.7283) (-0.747, -191.7283) (0.0866, -192.6768) (0.0866, -193.5401) knots 0 0 0 1 2 2 2
  spline S79 degree 2 poles (-0.5099, -193.5401) (-0.5099, -192.8732) (-0.9953, -192.2248) (-1.4436, -192.2248) knots 0 0 0 1 2 2 2
  spline S80 degree 2 poles (-1.4436, -192.2248) (-1.8919, -192.2248) (-2.381, -192.8732) (-2.381, -193.5401) knots 0 0 0 1 2 2 2
  spline S81 degree 2 poles (-2.381, -193.5401) (-2.381, -194.1885) (-1.8919, -194.8554) (-1.4436, -194.8554) knots 0 0 0 1 2 2 2
  spline S82 degree 2 poles (-1.4436, -194.8554) (-0.999, -194.8554) (-0.5099, -194.1996) (-0.5099, -193.5401) knots 0 0 0 1 2 2 2
  spline S83 degree 2 poles (1.7168, -195.3222) (1.2463, -195.3222) (0.7164, -194.785) (0.7164, -194.2033) knots 0 0 0 1 2 2 2
  line L67 (0.7164, -194.2033) -> (0.7164, -192.3026)
  line L68 (0.7164, -192.3026) -> (0.3274, -192.3026)
  line L69 (0.3274, -192.3026) -> (0.3274, -191.8246)
  line L70 (0.3274, -191.8246) -> (0.7164, -191.8246)
  line L71 (0.7164, -191.8246) -> (0.7164, -190.8391)
  line L72 (0.7164, -190.8391) -> (1.2944, -190.8391)
  line L73 (1.2944, -190.8391) -> (1.2944, -191.8246)
  line L74 (1.2944, -191.8246) -> (2.3578, -191.8246)
  line L75 (2.3578, -191.8246) -> (2.3578, -192.3026)
  line L76 (2.3578, -192.3026) -> (1.2944, -192.3026)
  line L77 (1.2944, -192.3026) -> (1.2944, -193.9365)
  spline S84 degree 2 poles (1.2944, -193.9365) (1.2944, -194.1959) (1.3129, -194.4811) (1.3759, -194.6034) knots 0 0 0 1 2 2 2
  spline S85 degree 2 poles (1.3759, -194.6034) (1.4278, -194.7109) (1.6612, -194.8183) (1.8613, -194.8183) knots 0 0 0 1 2 2 2
  spline S86 degree 2 poles (1.8613, -194.8183) (2.0021, -194.8183) (2.2651, -194.7331) (2.3244, -194.7072) knots 0 0 0 1 2 2 2
  line L78 (2.3244, -194.7072) -> (2.3578, -194.7072)
  line L79 (2.3578, -194.7072) -> (2.3578, -195.2259)
  spline S87 degree 2 poles (2.3578, -195.2259) (2.1947, -195.2703) (1.8613, -195.3222) (1.7168, -195.3222) knots 0 0 0 1 2 2 2
  spline S88 degree 2 poles (3.8212, -195.3222) (3.3507, -195.3222) (2.8209, -194.785) (2.8209, -194.2033) knots 0 0 0 1 2 2 2
  line L80 (2.8209, -194.2033) -> (2.8209, -192.3026)
  line L81 (2.8209, -192.3026) -> (2.4319, -192.3026)
  line L82 (2.4319, -192.3026) -> (2.4319, -191.8246)
  line L83 (2.4319, -191.8246) -> (2.8209, -191.8246)
  line L84 (2.8209, -191.8246) -> (2.8209, -190.8391)
  line L85 (2.8209, -190.8391) -> (3.3989, -190.8391)
  line L86 (3.3989, -190.8391) -> (3.3989, -191.8246)
  line L87 (3.3989, -191.8246) -> (4.4622, -191.8246)
  line L88 (4.4622, -191.8246) -> (4.4622, -192.3026)
  line L89 (4.4622, -192.3026) -> (3.3989, -192.3026)
  line L90 (3.3989, -192.3026) -> (3.3989, -193.9365)
  spline S89 degree 2 poles (3.3989, -193.9365) (3.3989, -194.1959) (3.4174, -194.4811) (3.4804, -194.6034) knots 0 0 0 1 2 2 2
  spline S90 degree 2 poles (3.4804, -194.6034) (3.5323, -194.7109) (3.7657, -194.8183) (3.9657, -194.8183) knots 0 0 0 1 2 2 2
  spline S91 degree 2 poles (3.9657, -194.8183) (4.1065, -194.8183) (4.3696, -194.7331) (4.4289, -194.7072) knots 0 0 0 1 2 2 2
  line L91 (4.4289, -194.7072) -> (4.4622, -194.7072)
  line L92 (4.4622, -194.7072) -> (4.4622, -195.2259)
  spline S92 degree 2 poles (4.4622, -195.2259) (4.2992, -195.2703) (3.9657, -195.3222) (3.8212, -195.3222) knots 0 0 0 1 2 2 2
  spline S93 degree 2 poles (7.7078, -193.5401) (7.7078, -194.407) (6.8742, -195.3518) (6.1776, -195.3518) knots 0 0 0 1 2 2 2
  spline S94 degree 2 poles (6.1776, -195.3518) (5.4626, -195.3518) (4.6438, -194.3774) (4.6438, -193.5401) knots 0 0 0 1 2 2 2
  spline S95 degree 2 poles (4.6438, -193.5401) (4.6438, -192.6805) (5.4885, -191.7283) (6.1776, -191.7283) knots 0 0 0 1 2 2 2
  spline S96 degree 2 poles (6.1776, -191.7283) (6.8742, -191.7283) (7.7078, -192.6768) (7.7078, -193.5401) knots 0 0 0 1 2 2 2
  spline S97 degree 2 poles (7.1113, -193.5401) (7.1113, -192.8732) (6.626, -192.2248) (6.1776, -192.2248) knots 0 0 0 1 2 2 2
  spline S98 degree 2 poles (6.1776, -192.2248) (5.7293, -192.2248) (5.2403, -192.8732) (5.2403, -193.5401) knots 0 0 0 1 2 2 2
  spline S99 degree 2 poles (5.2403, -193.5401) (5.2403, -194.1885) (5.7293, -194.8554) (6.1776, -194.8554) knots 0 0 0 1 2 2 2
  spline S100 degree 2 poles (6.1776, -194.8554) (6.6222, -194.8554) (7.1113, -194.1996) (7.1113, -193.5401) knots 0 0 0 1 2 2 2
  line L93 (12.1909, -195.2555) -> (12.1909, -193.2696)
  spline S101 degree 2 poles (12.1909, -193.2696) (12.1909, -193.0325) (12.1538, -192.6286) (12.0946, -192.5175) knots 0 0 0 1 2 2 2
  spline S102 degree 2 poles (12.0946, -192.5175) (12.0353, -192.3952) (11.8093, -192.2767) (11.6129, -192.2767) knots 0 0 0 1 2 2 2
  spline S103 degree 2 poles (11.6129, -192.2767) (11.4351, -192.2767) (11.0275, -192.4953) (10.8126, -192.7027) knots 0 0 0 1 2 2 2
  spline S104 degree 2 poles (10.8126, -192.7027) (10.8163, -192.7546) (10.8237, -192.8991) (10.8237, -192.9954) knots 0 0 0 1 2 2 2
  line L94 (10.8237, -192.9954) -> (10.8237, -195.2555)
  line L95 (10.8237, -195.2555) -> (10.2458, -195.2555)
  line L96 (10.2458, -195.2555) -> (10.2458, -193.2696)
  spline S105 degree 2 poles (10.2458, -193.2696) (10.2458, -193.0325) (10.2087, -192.6286) (10.1494, -192.5175) knots 0 0 0 1 2 2 2
  spline S106 degree 2 poles (10.1494, -192.5175) (10.0902, -192.3952) (9.8641, -192.2767) (9.6678, -192.2767) knots 0 0 0 1 2 2 2
  spline S107 degree 2 poles (9.6678, -192.2767) (9.4825, -192.2767) (9.0713, -192.5101) (8.8786, -192.6916) knots 0 0 0 1 2 2 2
  line L97 (8.8786, -192.6916) -> (8.8786, -195.2555)
  line L98 (8.8786, -195.2555) -> (8.3006, -195.2555)
  line L99 (8.3006, -195.2555) -> (8.3006, -191.8246)
  line L100 (8.3006, -191.8246) -> (8.8786, -191.8246)
  line L101 (8.8786, -191.8246) -> (8.8786, -192.2026)
  spline S108 degree 2 poles (8.8786, -192.2026) (9.1046, -191.9766) (9.5492, -191.7283) (9.816, -191.7283) knots 0 0 0 1 2 2 2
  spline S109 degree 2 poles (9.816, -191.7283) (10.1198, -191.7283) (10.5903, -192.0062) (10.7126, -192.3211) knots 0 0 0 1 2 2 2
  spline S110 degree 2 poles (10.7126, -192.3211) (10.9757, -192.0284) (11.4721, -191.7283) (11.7611, -191.7283) knots 0 0 0 1 2 2 2
  spline S111 degree 2 poles (11.7611, -191.7283) (11.9834, -191.7283) (12.3465, -191.8654) (12.4799, -192.021) knots 0 0 0 1 2 2 2
  spline S112 degree 2 poles (12.4799, -192.021) (12.617, -192.1766) (12.7689, -192.6435) (12.7689, -192.9954) knots 0 0 0 1 2 2 2
  line L102 (12.7689, -192.9954) -> (12.7689, -195.2555)
  line L103 (12.7689, -195.2555) -> (12.1909, -195.2555)
  line L104 (16.6406, -196.1743) -> (13.1135, -196.1743)
  line L105 (13.1135, -196.1743) -> (13.1135, -195.7779)
  line L106 (13.1135, -195.7779) -> (16.6406, -195.7779)
  line L107 (16.6406, -195.7779) -> (16.6406, -196.1743)
  line L108 (19.7047, -191.8246) -> (18.4116, -195.2555)
  line L109 (18.4116, -195.2555) -> (17.8929, -195.2555)
  line L110 (17.8929, -195.2555) -> (16.611, -191.8246)
  line L111 (16.611, -191.8246) -> (17.2371, -191.8246)
  line L112 (17.2371, -191.8246) -> (18.1745, -194.4663)
  line L113 (18.1745, -194.4663) -> (19.1045, -191.8246)
  line L114 (19.1045, -191.8246) -> (19.7047, -191.8246)
  spline S113 degree 2 poles (22.9021, -192.9695) (22.9021, -194.1996) (22.1871, -195.3518) (21.4423, -195.3518) knots 0 0 0 1 2 2 2
  spline S114 degree 2 poles (21.4423, -195.3518) (20.6865, -195.3518) (19.9789, -194.1773) (19.9789, -192.9732) knots 0 0 0 1 2 2 2
  spline S115 degree 2 poles (19.9789, -192.9732) (19.9789, -191.7357) (20.6939, -190.5909) (21.4423, -190.5909) knots 0 0 0 1 2 2 2
  spline S116 degree 2 poles (21.4423, -190.5909) (22.1945, -190.5909) (22.9021, -191.7765) (22.9021, -192.9695) knots 0 0 0 1 2 2 2
  spline S117 degree 2 poles (22.1167, -194.3626) (22.2056, -194.1366) (22.2797, -193.44) (22.2797, -192.9695) knots 0 0 0 1 2 2 2
  spline S118 degree 2 poles (22.2797, -192.9695) (22.2797, -192.499) (22.2056, -191.8061) (22.113, -191.5727) knots 0 0 0 1 2 2 2
  spline S119 degree 2 poles (22.113, -191.5727) (22.0203, -191.3393) (21.698, -191.0985) (21.4423, -191.0985) knots 0 0 0 1 2 2 2
  spline S120 degree 2 poles (21.4423, -191.0985) (21.1867, -191.0985) (20.857, -191.3393) (20.7606, -191.5801) knots 0 0 0 1 2 2 2
  spline S121 degree 2 poles (20.7606, -191.5801) (20.668, -191.8135) (20.6013, -192.5249) (20.6013, -192.9732) knots 0 0 0 1 2 2 2
  spline S122 degree 2 poles (20.6013, -192.9732) (20.6013, -193.4549) (20.6606, -194.0995) (20.7569, -194.3515) knots 0 0 0 1 2 2 2
  spline S123 degree 2 poles (20.7569, -194.3515) (20.8458, -194.5886) (21.1756, -194.8442) (21.4423, -194.8442) knots 0 0 0 1 2 2 2
  spline S124 degree 2 poles (21.4423, -194.8442) (21.6943, -194.8442) (22.024, -194.6034) (22.1167, -194.3626) knots 0 0 0 1 2 2 2
  line L115 (24.4693, -195.2555) -> (23.7358, -195.2555)
  line L116 (23.7358, -195.2555) -> (23.7358, -194.3811)
  line L117 (23.7358, -194.3811) -> (24.4693, -194.3811)
  line L118 (24.4693, -194.3811) -> (24.4693, -195.2555)
  line L119 (28.2114, -195.2555) -> (25.3919, -195.2555)
  line L120 (25.3919, -195.2555) -> (25.3919, -194.6071)
  spline S125 degree 2 poles (25.3919, -194.6071) (25.6957, -194.3218) (26.2366, -193.792) (26.496, -193.5067) knots 0 0 0 1 2 2 2
  spline S126 degree 2 poles (26.496, -193.5067) (27.0184, -192.9324) (27.4, -192.2433) (27.4, -191.8765) knots 0 0 0 1 2 2 2
  spline S127 degree 2 poles (27.4, -191.8765) (27.4, -191.6839) (27.2815, -191.3949) (27.174, -191.3022) knots 0 0 0 1 2 2 2
  spline S128 degree 2 poles (27.174, -191.3022) (27.0666, -191.2096) (26.785, -191.117) (26.6146, -191.117) knots 0 0 0 1 2 2 2
  spline S129 degree 2 poles (26.6146, -191.117) (26.4515, -191.117) (26.1181, -191.1985) (25.9662, -191.2615) knots 0 0 0 1 2 2 2
  spline S130 degree 2 poles (25.9662, -191.2615) (25.8365, -191.3134) (25.5957, -191.4616) (25.5216, -191.5134) knots 0 0 0 1 2 2 2
  line L121 (25.5216, -191.5134) -> (25.4882, -191.5134)
  line L122 (25.4882, -191.5134) -> (25.4882, -190.8613)
  spline S131 degree 2 poles (25.4882, -190.8613) (25.6772, -190.7687) (26.3552, -190.5872) (26.659, -190.5872) knots 0 0 0 1 2 2 2
  spline S132 degree 2 poles (26.659, -190.5872) (27.3, -190.5872) (28.0225, -191.2652) (28.0225, -191.8432) knots 0 0 0 1 2 2 2
  spline S133 degree 2 poles (28.0225, -191.8432) (28.0225, -192.1136) (27.8965, -192.5656) (27.7853, -192.7583) knots 0 0 0 1 2 2 2
  spline S134 degree 2 poles (27.7853, -192.7583) (27.6742, -192.9584) (27.3519, -193.3511) (27.174, -193.5401) knots 0 0 0 1 2 2 2
  spline S135 degree 2 poles (27.174, -193.5401) (26.885, -193.855) (26.1774, -194.5293) (25.9662, -194.7257) knots 0 0 0 1 2 2 2
  line L123 (25.9662, -194.7257) -> (28.2114, -194.7257)
  line L124 (28.2114, -194.7257) -> (28.2114, -195.2555)
  line L125 (29.8046, -195.2555) -> (29.071, -195.2555)
  line L126 (29.071, -195.2555) -> (29.071, -194.3811)
  line L127 (29.071, -194.3811) -> (29.8046, -194.3811)
  line L128 (29.8046, -194.3811) -> (29.8046, -195.2555)
  line L129 (33.5467, -195.2555) -> (30.7271, -195.2555)
  line L130 (30.7271, -195.2555) -> (30.7271, -194.6071)
  spline S136 degree 2 poles (30.7271, -194.6071) (31.0309, -194.3218) (31.5719, -193.792) (31.8312, -193.5067) knots 0 0 0 1 2 2 2
  spline S137 degree 2 poles (31.8312, -193.5067) (32.3536, -192.9324) (32.7353, -192.2433) (32.7353, -191.8765) knots 0 0 0 1 2 2 2
  spline S138 degree 2 poles (32.7353, -191.8765) (32.7353, -191.6839) (32.6167, -191.3949) (32.5093, -191.3022) knots 0 0 0 1 2 2 2
  spline S139 degree 2 poles (32.5093, -191.3022) (32.4018, -191.2096) (32.1202, -191.117) (31.9498, -191.117) knots 0 0 0 1 2 2 2
  spline S140 degree 2 poles (31.9498, -191.117) (31.7868, -191.117) (31.4533, -191.1985) (31.3014, -191.2615) knots 0 0 0 1 2 2 2
  spline S141 degree 2 poles (31.3014, -191.2615) (31.1717, -191.3134) (30.9309, -191.4616) (30.8568, -191.5134) knots 0 0 0 1 2 2 2
  line L131 (30.8568, -191.5134) -> (30.8235, -191.5134)
  line L132 (30.8235, -191.5134) -> (30.8235, -190.8613)
  spline S142 degree 2 poles (30.8235, -190.8613) (31.0124, -190.7687) (31.6904, -190.5872) (31.9943, -190.5872) knots 0 0 0 1 2 2 2
  spline S143 degree 2 poles (31.9943, -190.5872) (32.6352, -190.5872) (33.3577, -191.2652) (33.3577, -191.8432) knots 0 0 0 1 2 2 2
  spline S144 degree 2 poles (33.3577, -191.8432) (33.3577, -192.1136) (33.2317, -192.5656) (33.1206, -192.7583) knots 0 0 0 1 2 2 2
  spline S145 degree 2 poles (33.1206, -192.7583) (33.0094, -192.9584) (32.6871, -193.3511) (32.5093, -193.5401) knots 0 0 0 1 2 2 2
  spline S146 degree 2 poles (32.5093, -193.5401) (32.2203, -193.855) (31.5126, -194.5293) (31.3014, -194.7257) knots 0 0 0 1 2 2 2
  line L133 (31.3014, -194.7257) -> (33.5467, -194.7257)
  line L134 (33.5467, -194.7257) -> (33.5467, -195.2555)
  spline S147 degree 2 poles (2.2948, -201.3012) (2.2948, -201.6531) (2.0614, -202.2497) (1.865, -202.4497) knots 0 0 0 1 2 2 2
  spline S148 degree 2 poles (1.865, -202.4497) (1.6612, -202.6609) (1.1499, -202.8795) (0.8424, -202.8795) knots 0 0 0 1 2 2 2
  spline S149 degree 2 poles (0.8424, -202.8795) (0.5349, -202.8795) (0.0273, -202.672) (-0.1654, -202.4645) knots 0 0 0 1 2 2 2
  spline S150 degree 2 poles (-0.1654, -202.4645) (-0.4025, -202.2163) (-0.6692, -201.3827) (-0.6692, -200.7751) knots 0 0 0 1 2 2 2
  spline S151 degree 2 poles (-0.6692, -200.7751) (-0.6692, -200.1785) (-0.4247, -199.2189) (-0.1691, -198.8633) knots 0 0 0 1 2 2 2
  spline S152 degree 2 poles (-0.1691, -198.8633) (0.0792, -198.515) (0.8646, -198.126) (1.3796, -198.126) knots 0 0 0 1 2 2 2
  spline S153 degree 2 poles (1.3796, -198.126) (1.5315, -198.126) (1.7983, -198.1556) (1.8983, -198.1889) knots 0 0 0 1 2 2 2
  line L135 (1.8983, -198.1889) -> (1.8983, -198.778)
  line L136 (1.8983, -198.778) -> (1.8724, -198.778)
  spline S154 degree 2 poles (1.8724, -198.778) (1.7872, -198.7336) (1.476, -198.6558) (1.2981, -198.6558) knots 0 0 0 1 2 2 2
  spline S155 degree 2 poles (1.2981, -198.6558) (0.7276, -198.6558) (0.0273, -199.4264) (-0.0394, -200.1822) knots 0 0 0 1 2 2 2
  spline S156 degree 2 poles (-0.0394, -200.1822) (0.1792, -200.0303) (0.6386, -199.8636) (0.9128, -199.8636) knots 0 0 0 1 2 2 2
  spline S157 degree 2 poles (0.9128, -199.8636) (1.1796, -199.8636) (1.5797, -199.9711) (1.7983, -200.1341) knots 0 0 0 1 2 2 2
  spline S158 degree 2 poles (1.7983, -200.1341) (2.0502, -200.323) (2.2948, -200.9084) (2.2948, -201.3012) knots 0 0 0 1 2 2 2
  spline S159 degree 2 poles (1.6723, -201.3271) (1.6723, -201.0455) (1.5241, -200.6639) (1.3611, -200.5305) knots 0 0 0 1 2 2 2
  spline S160 degree 2 poles (1.3611, -200.5305) (1.2388, -200.4342) (0.935, -200.3712) (0.7757, -200.3712) knots 0 0 0 1 2 2 2
  spline S161 degree 2 poles (0.7757, -200.3712) (0.5608, -200.3712) (0.157, -200.5009) (-0.0394, -200.6231) knots 0 0 0 1 2 2 2